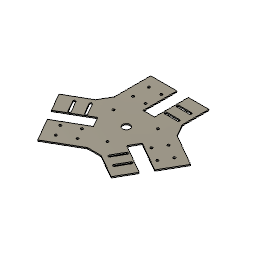
Robot Delta base v4 (Autodesk Fusion 360 design; units mm, degrees)
Autodesk Fusion 360 part; units mm, degrees
sketch "Boceto1" plane through (0, 0, 0) normal (0, 0, 1) x (1, 0, 0)
  circle A0 centre (0, 0) radius 100
  line L0 (0, 200.0885) -> (-173.2817, -100.0442)
  line L1 (-173.2817, -100.0442) -> (173.2817, -100.0442)
  line L2 (173.2817, -100.0442) -> (0, 200.0885)
  line L3 (0, -100.0442) -> (0, 200.0885) construction
  line L4 (-173.2817, -100.0442) -> (86.6408, 50.0221) construction
  line L5 (173.2817, -100.0442) -> (-86.6408, 50.0221) construction
  line L6 (51.9615, -30) -> (59.4615, -17.0096)
  line L7 (59.4615, -17.0096) -> (128.7436, -57.0096)
  line L8 (44.4615, -42.9904) -> (113.7436, -82.9904)
  line L9 (51.9615, -30) -> (44.4615, -42.9904)
  line L10 (-15, 60) -> (-15, 140)
  line L11 (0.5917, 60) -> (15, 60)
  line L12 (15, 60) -> (15, 140)
  line L13 (-123.1844, 140) -> (49.0279, 140)
  line L14 (-15, 60) -> (0.5917, 60)
  line L15 (157.2934, 41.8591) -> (75.3655, -100.0442)
  line L16 (-44.4615, -42.9904) -> (-113.7436, -82.9904)
  line L17 (-59.4615, -17.0096) -> (-128.7436, -57.0096)
  line L18 (-30.9577, -176.4773) -> (-124.184, -15.0046)
  line L19 (-44.4615, -42.9904) -> (-59.4615, -17.0096)
  circle A1 centre (0, 0) radius 10
  line L20 (-115.5498, 0.1381) -> (-24.8334, -156.9872) construction
  line L21 (212.8999, -69.8468) -> (210.5798, -60.2903) construction
  line L22 (57.7095, -100.0442) -> (164.8904, 85.5986) construction
  line L23 (57.7861, 100) -> (-125, 100) construction
  line L24 (-85, 150) -> (-15, 150)
  line L25 (-15, 150) -> (-15, 50)
  line L26 (-15, 50) -> (-85, 50)
  line L27 (-85, 50) -> (-85, 150)
  circle A2 centre (45, 84) radius 3
  circle A3 centre (25, 84) radius 3
  circle A4 centre (25, 116) radius 3
  circle A5 centre (45, 116) radius 3
  line L28 (28.8663, 150.0905) -> (70, 150.0905)
  line L29 (70, 150.0905) -> (70, 78.8449)
  line L30 (21, 113) -> (55, 113)
  line L31 (21, 119) -> (55, 119)
  arc A6 (55, 113) -> (55, 119) centre (55, 116) ccw
  arc A7 (21, 119) -> (21, 113) centre (21, 116) ccw
  line L32 (21, 81) -> (55, 81)
  circle A8 centre (25, 84) radius 3
  circle A9 centre (45, 84) radius 3
  line L33 (21, 87) -> (55, 87)
  arc A10 (21, 87) -> (21, 81) centre (21, 84) ccw
  arc A11 (55, 81) -> (55, 87) centre (55, 84) ccw
  line L34 (-0.8013, -98.6122) -> (-87.4038, -148.6122)
  line L35 (-35.8013, -37.9904) -> (-0.8013, -98.6122)
  line L36 (-44.4615, -42.9904) -> (-113.7436, -82.9904)
  line L37 (-122.4038, -87.9904) -> (-35.8013, -37.9904)
  line L38 (-87.4038, -148.6122) -> (-122.4038, -87.9904)
  line L39 (-59.6514, -176.6808) -> (-145.7575, -27.5406)
  line L40 (-59.4615, -17.0096) -> (-128.7436, -57.0096)
  line L41 (-52.2574, -29.4875) -> (-59.4615, -17.0096)
  line L42 (-44.4615, -42.9904) -> (-52.2574, -29.4875)
  line L43 (-80.6481, -22.3135) -> (-97.6481, 7.1314)
  circle A12 centre (-112.9589, -36.3494) radius 3
  circle A13 centre (-122.9589, -19.0289) radius 3
  circle A14 centre (-85.2461, -20.3494) radius 3
  circle A15 centre (-95.2461, -3.0289) radius 3
  line L44 (-85.8442, -25.3135) -> (-102.8442, 4.1314)
  arc A16 (-85.8442, -25.3135) -> (-80.6481, -22.3135) centre (-83.2461, -23.8135) ccw
  arc A17 (-97.6481, 7.1314) -> (-102.8442, 4.1314) centre (-100.2461, 5.6314) ccw
  arc A18 (-113.557, -41.3135) -> (-108.3609, -38.3135) centre (-110.9589, -39.8135) ccw
  line L45 (-108.3609, -38.3135) -> (-125.3609, -8.8686)
  line L46 (-113.557, -41.3135) -> (-130.557, -11.8686)
  arc A19 (-125.3609, -8.8686) -> (-130.557, -11.8686) centre (-127.9589, -10.3686) ccw
  line L47 (-144.4154, -50.0463) -> (-164.9822, -14.4235)
  line L48 (-164.9822, -14.4235) -> (-103.2817, 21.1993)
  line L49 (85.8013, 48.6122) -> (172.4038, -1.3878)
  line L50 (50.8013, -12.0096) -> (85.8013, 48.6122)
  line L51 (59.4615, -17.0096) -> (128.7436, -57.0096)
  line L52 (137.4038, -62.0096) -> (50.8013, -12.0096)
  line L53 (172.4038, -1.3878) -> (137.4038, -62.0096)
  line L54 (182.8357, 36.6808) -> (96.7296, -112.4594)
  line L55 (44.4615, -42.9904) -> (113.7436, -82.9904)
  line L56 (51.6657, -30.5125) -> (44.4615, -42.9904)
  line L57 (59.4615, -17.0096) -> (51.6657, -30.5125)
  line L58 (59.6481, -58.6865) -> (42.6481, -88.1314)
  circle A20 centre (87.9589, -79.6506) radius 3
  circle A21 centre (77.9589, -96.9711) radius 3
  circle A22 centre (60.2461, -63.6506) radius 3
  circle A23 centre (50.2461, -80.9711) radius 3
  line L59 (64.8442, -61.6865) -> (47.8442, -91.1314)
  arc A24 (64.8442, -61.6865) -> (59.6481, -58.6865) centre (62.2461, -60.1865) ccw
  arc A25 (42.6481, -88.1314) -> (47.8442, -91.1314) centre (45.2461, -89.6314) ccw
  arc A26 (92.557, -77.6865) -> (87.3609, -74.6865) centre (89.9589, -76.1865) ccw
  line L60 (87.3609, -74.6865) -> (70.3609, -104.1314)
  line L61 (92.557, -77.6865) -> (75.557, -107.1314)
  arc A27 (70.3609, -104.1314) -> (75.557, -107.1314) centre (72.9589, -105.6314) ccw
  line L62 (115.549, -100.0442) -> (94.9822, -135.667)
  line L63 (94.9822, -135.667) -> (33.2817, -100.0442)
  line L64 (-15, 150) -> (28.8663, 150.0905)
  line L65 (15, 150.0619) -> (15, 140)
  line L66 (-144.4154, -50.0463) -> (-122.4038, -87.9904)
  line L67 (115.549, -100.0442) -> (137.4038, -62.0096)
  line L68 (122.3417, -88.2227) -> (113.7436, -82.9904)
  line L69 (-137.4729, -62.0138) -> (-128.7436, -57.0096)
  circle A28 centre (118.8973, -36.3138) radius 3
  circle A29 centre (135.4123, -7.709) radius 3
  circle A30 centre (98.8228, 13.416) radius 3
  circle A31 centre (82.3078, -15.1888) radius 3
  circle A32 centre (-61.03, 121.125) radius 3
  circle A33 centre (-28, 121.125) radius 3
  circle A34 centre (-28, 78.875) radius 3
  circle A35 centre (-61.03, 78.875) radius 3
  circle A36 centre (-74.3823, -113.416) radius 3
  circle A37 centre (-90.8973, -84.8112) radius 3
  circle A38 centre (-54.3078, -63.6862) radius 3
  circle A39 centre (-37.7928, -92.291) radius 3
  line L70 (-3.1207, -99.9513) -> (33.2817, -100.0442)
  line L71 (-103.2817, 21.1993) -> (-85, 52.8641)
  line L72 (0, 0) -> (15.0803, -100.0442) construction
  circle A40 centre (8.9431, -59.3298) radius 3
  circle A41 centre (0, 0) radius 60 construction
  circle A42 centre (46.9095, 37.4099) radius 3
  circle A43 centre (-55.8526, 21.9199) radius 3
  point P0 (-86.6025, -50)
  point P1 (-85.2461, -20.3494)
  point P2 (60.2461, -63.6506)
  dimension "d1" = 200
  dimension "d5" = 80
  dimension "d6" = 60
  dimension "d7" = 30
  dimension "d8" = 80
  dimension "d9" = 30
  dimension "d10" = 15
  dimension "d13" = 60
  dimension "d16" = 80
  dimension "d17" = 30
  dimension "d18" = 15
  dimension "d19" = 60
  dimension "d22" = 80
  dimension "d24" = 80
  dimension "d25" = 20
  dimension "d27" = 70
  dimension "d28" = 100
  dimension "d29" = 50
  dimension "d47" = 6
  dimension "d48" = 6
  dimension "d49" = 6
  dimension "d50" = 6
  dimension "d51" = 20
  dimension "d52" = 20
  dimension "d53" = 32
  dimension "d55" = 10
  dimension "d56" = 10
  dimension "d57" = 16
  dimension "d58" = 16
  dimension "d59" = 32
  dimension "d60" = 10
  dimension "d61" = 4
  dimension "d62" = 4
  dimension "d63" = 10
  dimension "d68" = 6
  dimension "d69" = 13
  dimension "d70" = 21.125
  dimension "d71" = 6
  dimension "d72" = 33.03
  dimension "d73" = 21.125
  dimension "d74" = 21.125
  dimension "d76" = 360
  dimension "d94" = 36.4024
  dimension "d95" = 18.201
  dimension "d96" = 6
  dimension "d98" = 60
  dimension "d99" = 120
  dimension "d101" = 360
  constraint coincident A0.centre A1.centre
  constraint midpoint L1 L3.start
  constraint perpendicular L1 L3
  constraint midpoint L2 L4.end
  constraint perpendicular L2 L4
  constraint midpoint L0 L5.end
  constraint perpendicular L0 L5
  constraint coincident L5 L6.start
  constraint perpendicular L5 L6
  constraint perpendicular L6 L7
  constraint symmetric L5 L6.start L9.start
  constraint symmetric L5 L6.end L8.start
  constraint symmetric L5 L7.end L8.end
  constraint perpendicular L12 L13
  constraint perpendicular L3 L14
  constraint perpendicular L17 L18
  constraint perpendicular L17 L19
  constraint horizontal L13
  constraint coincident L0 L18.end
  constraint coincident L1 L15.end
  constraint coincident A0 P0
  constraint coincident L4 P0
  constraint perpendicular L4 L20
  constraint tangent A0 L20
  constraint perpendicular L5 L22
  constraint tangent A0 L22
  constraint coincident L1 L22.start
  constraint equal L10 L12
  constraint coincident L2 L23.start
  constraint perpendicular L12 L23
  constraint horizontal L24
  constraint vertical L25
  constraint horizontal L26
  constraint vertical L27
  constraint coincident L2 L28.start
  constraint parallel L13 L28
  constraint coincident L2 L29.end
  constraint perpendicular L28 L29
  constraint perpendicular L3 L30
  constraint tangent A4 L31
  constraint tangent L30 A6
  constraint tangent L31 A6
  constraint tangent L30 A7
  constraint symmetric L23 A4 A8
  constraint symmetric L23 A5 A9
  constraint symmetric L23 L30.start L33.start
  constraint symmetric L23 L30.end L33.end
  constraint symmetric L23 L31.start L32.start
  constraint symmetric L23 L31.end L32.end
  constraint symmetric L23 A6 A11
  constraint symmetric L23 A7 A10
  constraint coincident L64 L65.start
  constraint perpendicular L13 L65
  constraint coincident L67 L68.start
  constraint coincident L66 L69.start
  constraint symmetric L22 A28 A31
  constraint symmetric L22 A29 A30
  constraint coincident A0 L70.start
  constraint coincident L34 L70.start
  constraint coincident L0 L71.end
  constraint coincident L27 L71.end
  constraint parallel L0 L71
  constraint coincident L1 L72.end
  constraint coincident L72 A40.centre
  constraint concentric A1 A41
  measures "d1" diameter of A0
  measures "d5" distance of L6.end L7.end
  measures "d6" distance of A0.centre L6.start
  measures "d7" distance of L7 L8
  measures "d8" distance of L10.start L10.end
  measures "d9" distance of L10 L12
  measures "d10" distance of L3 L12
  measures "d13" distance of A0.centre L14
  measures "d16" distance of L16.start L16.end
  measures "d17" distance of L16 L17
  measures "d18" distance of L4 L17
  measures "d19" distance of A0.centre L19
  measures "d22" distance of L17.start L17.end
  measures "d24" distance of L11 L13
  measures "d25" diameter of A1
  measures "d27" distance of L25 L27
  measures "d28" distance of L24.start L26.end
  measures "d29" distance of L23 L24
  measures "d47" diameter of A2
  measures "d48" diameter of A3
  measures "d49" diameter of A4
  measures "d50" diameter of A5
  measures "d51" distance of A2.centre A3.centre
  measures "d52" horizontal distance of A4.centre A5.centre
  measures "d53" vertical distance of A2.centre A5.centre
  measures "d55" distance of L12 A3.centre
  measures "d56" distance of L12 A4.centre
  measures "d57" distance of L23 A5.centre
  measures "d58" distance of L23 A4.centre
  measures "d59" distance of A3.centre A4.centre
  measures "d60" horizontal distance of A5.centre L30.end
  measures "d61" horizontal distance of A4.centre L30.start
  measures "d62" horizontal distance of A4.centre L31.start
  measures "d63" horizontal distance of A5.centre L31.end
  measures "d68" diameter of A28
  measures "d69" distance of L7 A28.centre
  measures "d70" distance of L22 A28.centre
  measures "d71" diameter of A29
  measures "d72" distance of A28.centre A29.centre
  measures "d73" distance of L22 A29.centre
  measures "d74" distance of L22 A30.centre
  measures "d94" horizontal distance of L63.end L70.start
  measures "d95" horizontal distance of L70.start L72.end
  measures "d96" diameter of A40
  measures "d98" distance of A0.centre A40.centre
  measures "d99" diameter of A41
extrude "Extruir3" add sketch "Boceto1" along normal blind 3 contours A0 L7 L49 L50 L51 L52 A30 | A0 L2 L7 L15 L49 L51 L52 A30 | A0 L1 L8 L15 L55 L59 A25 A26 L60 L70 | A0 L6 L8 L9 L11 L12 L14 L17 L19 L25 L26 L27 L32 L33 A10 A11 L34 L35 L37 L40 L41 L42 L43 L44 A16 A17 L49 L50 L52 L55 L56 L57 L58 L59 A24 A25 L70 | L2 L7 L15 L51 L52 L54 | A0 L2 L12 L13 L30 L31 A7 L33 A11 L49 | L1 L8 L15 L54 L55 A26 L61 | L2 L52 L53 L54 | L2 L15 L49 L54 | L2 L15 L49 | L1 L54 L67 L68 | L2 L49 L53 L54 | L2 L28 L29 L30 L31 A6 | L1 L60 L61 A27 L62 L63 | A0 L1 L16 L18 L34 L36 L37 A39 | A0 L16 L34 L35 L36 L37 A39 | A0 L10 L25 L26 L27 A35 | A0 L0 L10 L13 L25 L27 A35 | L2 L13 L64 L65 | L1 L18 L34 | L0 L13 L24 L25 | L1 L18 L34 L39 | L1 L16 L18 L36 L37 L39 | L0 L13 L24 L27 | L0 L13 L27 | L1 L34 L38 L39 | L1 L37 L38 L39 | A0 L0 L17 L18 L27 L40 L44 A17 A18 L45 L71 | L0 L17 L18 L39 L40 A18 L46 | L0 L45 L46 A19 L47 L48 | L0 L39 L66 L69
